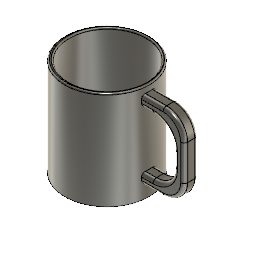
Mug v2 (Autodesk Fusion 360 design; units mm, degrees)
Autodesk Fusion 360 part; units mm, degrees
sketch "Boceto1" plane through (0, 0, 0) normal (0, 1, 0) x (1, 0, 0)
  line L0 (0, 0) -> (60, 0)
  line L1 (60, 0) -> (60, -70)
  line L2 (60, -70) -> (0, -70)
  line L3 (0, -70) -> (0, 0)
  line L4 (60, -11.9216) -> (60, -60)
  line L5 (60, -10) -> (90, -10)
  line L6 (90, -10) -> (90, -65)
  line L7 (90, -65) -> (60, -65)
  line L8 (60, -65) -> (60, -10)
  line L9 (60, -57.5606) -> (82.8089, -57.5606)
  line L10 (82.8089, -57.5606) -> (82.8089, -17.017)
  line L11 (82.8089, -17.017) -> (60, -17.017)
  line L12 (60, -17.017) -> (60, -57.5606)
  dimension "d1" = 60
  dimension "d2" = 70
  dimension "d3" = 30
  dimension "d4" = 55
  constraint horizontal L0
  constraint vertical L1
  constraint horizontal L2
  constraint vertical L3
  constraint coincident L0.start L3.end
  constraint vertical L4
  constraint coincident L1 L4.end
  constraint horizontal L5
  constraint vertical L6
  constraint horizontal L7
  constraint vertical L8
  constraint coincident L1 L5.start
  constraint horizontal L9
  constraint vertical L10
  constraint horizontal L11
  constraint vertical L12
  constraint coincident L8 L9.start
  measures "d1" distance of L0.start L0.end
  measures "d2" distance of L0.start L2.end
  measures "d3" distance of L5.start L5.end
  measures "d4" distance of L5.start L7.end
extrude "Extruir1" add sketch "Boceto1" along normal blind 60 contours L0 L1 L2 L3 L4 L8 L12 | L1 L4 L5 L6 L7 L8 L9 L10 L11
sketch "Boceto3" plane through (0, 0, 65) normal (0, 0, 1) x (-1, 0, 0)
  line L0 (-60, 0) -> (-90, 0)
  line L1 (-90, 0) -> (-90, -60)
  line L2 (-90, -60) -> (-60, -60)
  line L3 (-60, -60) -> (-60, 0)
  line L4 (-60, -60) -> (-90, -60)
  line L5 (-90, -60) -> (-90, -35)
  line L6 (-90, -35) -> (-60, -35)
  line L7 (-60, -35) -> (-60, -60)
  line L8 (-60, 0) -> (-90, 0)
  line L9 (-90, 0) -> (-90, -25)
  line L10 (-90, -25) -> (-60, -25)
  line L11 (-60, -25) -> (-60, 0)
  dimension "d7" = 25
  dimension "d8" = 25
  constraint horizontal L4
  constraint vertical L5
  constraint horizontal L6
  constraint vertical L7
  constraint coincident L1 L5.end
  constraint coincident L2.end L3.start
  constraint horizontal L8
  constraint vertical L9
  constraint horizontal L10
  constraint vertical L11
  constraint coincident L0.start L3.end
  measures "d7" distance of L2.end L6.end
  measures "d8" distance of L0.start L10.end
extrude "Extruir2" cut sketch "Boceto3" against normal blind 65 contours L1 L2 L3 L4 L5 L6 L7
sketch "Boceto4" plane through (0, 0, 65) normal (0, 0, 1) x (-1, 0, 0)
  line L0 (-90, -35) -> (-60, -35)
  line L1 (-60, -35) -> (-60, 0)
  line L2 (-60, 0) -> (-90, 0)
  line L3 (-90, 0) -> (-90, -35)
  line L4 (-90, 0) -> (-60, 0)
  line L5 (-60, 0) -> (-60, -25)
  line L6 (-60, -25) -> (-90, -25)
  line L7 (-90, -25) -> (-90, 0)
  dimension "d11" = 25
  constraint horizontal L4
  constraint vertical L5
  constraint horizontal L6
  constraint vertical L7
  constraint coincident L2.end L3.start
  measures "d11" distance of L2.end L6.end
extrude "Extruir3" cut sketch "Boceto4" against normal blind 95 contours L1 L2 L3 L4 L5 L6 L7
fillet "Empalme1" radius 30 4 edges at (60, 0, 35) (0, 0, 35) (60, 60, 35) (0, 60, 35)
sketch "Boceto5" plane through (0, 0, 0) normal (0, 0, 1) x (1, 0, 0)
hole "Agujero1" at (30.266, 30.2562, 70) direction (0, 0, -1) diameter 55 depth 52 tip angle 180
fillet "Empalme2" radius 15 4 edges at (90, 30, 65) (90, 30, 10) (82.8089, 30, 57.5606) (82.8089, 30, 17.017)
fillet "Empalme3" radius 2.5 20 edges at (63.6946, 25, 17.017) (78.4155, 25, 21.4104) (82.8089, 25, 37.2888) (78.4155, 25, 53.1672) (63.6946, 25, 57.5606) (67.2902, 25, 65) (85.6066, 25, 60.6066) (90, 25, 37.5) (85.6066, 25, 14.3934) (67.2902, 25, 10) (67.2902, 35, 10) (85.6066, 35, 14.3934) (90, 35, 37.5) (85.6066, 35, 60.6066) (67.2902, 35, 65) (63.6946, 35, 57.5606) (78.4155, 35, 53.1672) (82.8089, 35, 37.2888) (78.4155, 35, 21.4104) (63.6946, 35, 17.017)
fillet "Empalme4" radius 1 2 edges at (4.627, 40.2006, 70) (42.1066, 2.5513, 70)
